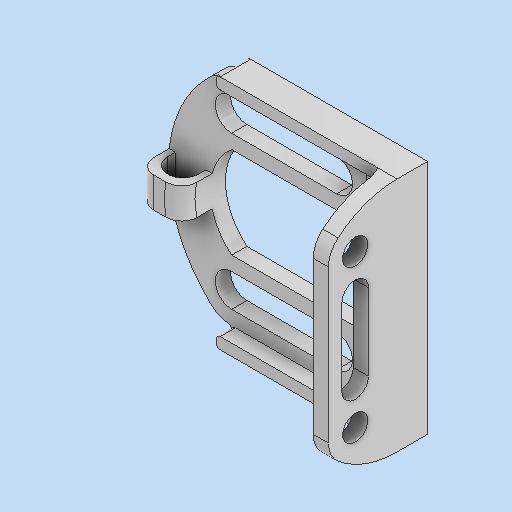
# Autodesk Inventor part: X-Gantry Enstop Mount
Saved by Autodesk Inventor 2023.2 (Build 272271000, 271)
## iProperties
Created: 2024-02-13
Part Number: X-Gantry Enstop Mount
Material: Generisch
Document SubType Name: Modeling
Designer: Nils Bade
Density: 1 g/cm^3
Appearance: Resin-3D-Druck
Description: Fertigung
Auf Bestellliste: True
Author: Nils Bade
Autodesk Inventor part; units mm, degrees
ref_plane "YZ Plane" through (0, 0, 0) normal (1, 0, 0) x (0, 1, 0)
sketch "S-Schiene" plane through (0, 0, 0) normal (0, 0, 1) x (1, 0, 0)
  line L0 (-30.84, 0) -> (5.14, 0)
  line L1 (0, -9.1) -> (0, 19.6)
  circle A0 centre (-8.51163, 10) radius 2.15 construction
  circle A1 centre (-8.51163, 10) radius 3.5 construction
  line L2 (-4, 10) -> (-21.7, 10) construction
  line L3 (-4, 12.15) -> (-21.7, 12.15)
  line L4 (-21.7, 7.85) -> (-4, 7.85)
  arc A2 (-4, 7.85) -> (-4, 12.15) centre (-4, 10) ccw
  arc A3 (-21.7, 12.15) -> (-21.7, 7.85) centre (-21.7, 10) ccw
  line L5 (-4, 10) -> (-21.7, 10) construction
  line L6 (0, 14) -> (-21.7, 14)
  line L7 (-21.7, 6) -> (0, 6)
  arc A4 (-4, 6) -> (-4, 14) centre (-4, 10) ccw construction
  arc A5 (-21.7, 14) -> (-21.7, 6) centre (-21.7, 10) ccw
  circle A6 centre (-7.766156, 0) radius 5 construction
  line L8 (-21.7, 10) -> (-8, 10) construction
  line L9 (-21.7, 7.849114) -> (-8, 7.849114)
  line L10 (-8, 12.150886) -> (-21.7, 12.150886)
  arc A7 (-21.7, 12.150886) -> (-21.7, 7.849114) centre (-21.7, 10) ccw
  arc A8 (-8, 7.849114) -> (-8, 12.150886) centre (-8, 10) ccw
  line L11 (0, 14) -> (-21.7, 14)
  line L12 (-21.7, 14) -> (-21.7, 15.5)
  line L13 (-21.7, 15.5) -> (0, 15.5)
  line L14 (0, 15.5) -> (0, 14)
  point P0 (-12.85, 10)
  point P1 (-12.85, 10)
  point P2 (0, 10)
  point P3 (-23.85, 10)
  point P4 (-1.85, 10)
  point P5 (0, 0)
  point P6 (-14.85, 10)
  point P7 (-7.938264, 12.15)
  point P8 (-7.938264, 7.85)
  point P9 (0, 15.5)
  dimension "d1" = 4.3
  dimension "d2" = 7
  dimension "d3" = 10
  dimension "d4" = 4.3
  dimension "d5" = 8
  dimension "d6" = 22
  dimension "d10" = 10
  dimension "d24" = 4
  dimension "d45" = 1.5
  constraints: 32 end point, 15 point on circle, 12 tangent, 9 centre point, 8 point on line, 6 equal length, 3 midpoint, 2 perpendicular, 1 coincident, 1 horizontal
  measures "d1" diameter of A0
  measures "d2" diameter of A1
  measures "d3" distance from line of A0.centre L0
  measures "d4" diameter of A3
  measures "d5" diameter of A5
  measures "d6" distance of point (-23.85, 10) point (-1.85, 10)
  measures "d10" diameter of A6
  measures "d24" distance of L2.start L8.end
  measures "d45" distance between parallel lines of L11 L13
sketch "S-Schiene outline for Ex-Schiene" plane through (0, 0, 0) normal (0, 0, 1) x (1, 0, 0)
  arc A0 (-21.7, 14) -> (-21.7, 6) centre (-21.7, 10) ccw
  line L0 (-21.7, 6) -> (0, 6)
  line L1 (0, 6) -> (0, 14)
  line L2 (0, 14) -> (-21.7, 14)
  line L3 (-21.7, 12.15) -> (-7.938264, 12.15)
  arc A1 (-7.938264, 12.15) -> (-7.938264, 7.85) centre (-8, 10) cw
  line L4 (-7.938264, 7.85) -> (-21.7, 7.85)
  arc A2 (-21.7, 7.85) -> (-21.7, 12.15) centre (-21.7, 10) cw
extrude "Ex-Schiene" add sketch "S-Schiene outline for Ex-Schiene" along normal blind 2
sketch "S-Schiene outline for Ex-Biegesteifigkeit" plane through (0, 0, 0) normal (0, 0, 1) x (1, 0, 0)
  line L0 (-21.7, 15.5) -> (-21.7, 14)
  line L1 (0, 15.5) -> (-21.7, 15.5)
  line L2 (0, 14) -> (0, 15.5)
  line L3 (-21.7, 14) -> (0, 14)
extrude "Ex-Biegesteifigkeit" add sketch "S-Schiene outline for Ex-Biegesteifigkeit" along normal blind 4
sketch "S-Front" plane through (0, 0, 0) normal (1, 0, 0) x (0, 1, 0)
  circle A0 centre (10, 9.5) radius 1.65
  circle A1 centre (10, 9.5) radius 3
  line L0 (6, 2) -> (14, 2) construction
  line L1 (0, 9.5) -> (5.032699, 9.5) construction
  line L2 (0, 7.75) -> (5.032699, 7.75)
  line L3 (5.032699, 11.25) -> (0, 11.25)
  arc A2 (0, 11.25) -> (0, 7.75) centre (0, 9.5) ccw construction
  arc A3 (5.032699, 7.75) -> (5.032699, 11.25) centre (5.032699, 9.5) ccw
  line L4 (0, 15.6) -> (0, -2.6)
  line L5 (0, 9.5) -> (10, 9.5) construction
  line L6 (0, 6) -> (10, 6) construction
  line L7 (10, 13) -> (0, 13)
  arc A4 (0, 13) -> (0, 6) centre (0, 9.5) ccw construction
  arc A5 (10, 6) -> (10, 13) centre (10, 9.5) ccw
  line L8 (14, 0) -> (14, 2)
  line L9 (6, 0) -> (14, 0)
  line L10 (6, 0) -> (6, 2)
  line L11 (6, 0) -> (0, 0)
  line L12 (14, 2) -> (6, 2)
  line L13 (15.5, 0) -> (15.5, 4)
  arc A6 (15.5, 4) -> (12.682482, 11.748175) centre (3.4375, 4) ccw
  line L14 (6, 0) -> (15.5, 0)
  line L15 (15.5, 0) -> (15.5, 4)
  line L16 (14, 4) -> (15.5, 4)
  line L17 (14, 2) -> (14, 4)
  line L18 (6, 2) -> (14, 2)
  line L19 (6, 0) -> (6, 2)
  point P0 (2.51635, 9.5)
  point P1 (5, 9.5)
  point P2 (0, 13)
  dimension "d11" = 3.3
  dimension "d13" = 6
  dimension "d15" = 3.5
  dimension "d16" = 7
  dimension "d23" = 9.5
  constraints: 18 end point, 11 point on circle, 10 tangent, 7 centre point, 2 coincident, 2 midpoint, 2 parallel, 1 perpendicular, 1 point on line
  measures "d11" diameter of A0
  measures "d13" diameter of A1
  measures "d15" diameter of A3
  measures "d16" diameter of A5
  measures "d23" distance from line of L9 A0.centre
sketch "S-Front outline for Ex-Front" plane through (0, 0, 0) normal (1, 0, 0) x (0, 1, 0)
  line L0 (6, 0) -> (14, 0)
  line L1 (0, 0) -> (6, 0)
  line L2 (14, 0) -> (15.5, 0)
  line L3 (0, 7.75) -> (0, 0)
  line L4 (15.5, 0) -> (15.5, 4)
  line L5 (5.032699, 7.75) -> (0, 7.75)
  arc A0 (15.5, 4) -> (12.682482, 11.748175) centre (3.4375, 4) ccw
  arc A1 (5.032699, 11.25) -> (5.032699, 7.75) centre (5.032699, 9.5) cw
  arc A2 (12.682482, 11.748175) -> (10, 13) centre (10, 9.5) ccw
  line L6 (0, 11.25) -> (5.032699, 11.25)
  line L7 (10, 13) -> (0, 13)
  line L8 (0, 13) -> (0, 11.25)
  circle A3 centre (10, 9.5) radius 1.65
extrude "Ex-Front" add sketch "S-Front outline for Ex-Front" along normal blind 2
fillet "Rundung-4mm" radius 4 2 edges at (0, 6, 1) (0, 10, 2)
extrude "Ex-SchraubenkopfEinlasss" [suppressed]
mirror "Spiegeln2" about plane through (0, 0, 0) normal (0, 1, 0)
ref_plane "E-Slide1" through (-21.7, 10, 0) normal (0, -1, 0) x (1, 0, 0)
ref_plane "E-slide2" through (-21.7, -10, 0) normal (0, -1, 0) x (1, 0, 0)
sketch "S-Extension" plane through (0, 0, 0) normal (0, 0, 1) x (1, 0, 0)
  arc A0 (-21.7, 14) -> (-21.7, 6) centre (-21.7, 10) ccw
  arc A1 (-21.7, -6) -> (-21.7, -14) centre (-21.7, -10) ccw
  arc A2 (-21.7, -6) -> (-21.7, -14) centre (-21.7, -10) ccw
  arc A3 (-21.7, 6) -> (-21.7, -6) centre (-16.705119, 0) ccw
  arc A4 (-21.7, 14) -> (-21.7, 6) centre (-21.7, 10) ccw
  arc A5 (-24.406352, 12.945447) -> (-24.445645, -12.908854) centre (-12.261257, -0.000191) ccw
  line L0 (-24.251564, 2) -> (-29.899061, 2)
  line L1 (-36.038087, 0) -> (6.006348, 0) construction
  line L2 (-29.899104, -2) -> (-24.251564, -2)
  point P0 (0, 0)
  point P1 (-24.484334, 12.871843)
  point P2 (-24.445645, -12.908854)
  dimension "d34" = 2
  dimension "d36" = 2
  constraints: 10 point on circle, 4 end point, 2 centre point, 2 horizontal, 1 tangent
  measures "d34" distance between parallel lines of L1 L0
  measures "d36" distance between parallel lines of L2 L1
sketch "S-Extension outline for Ex-Extension1" plane through (0, 0, 0) normal (0, 0, 1) x (1, 0, 0)
  arc A0 (-21.7, -6) -> (-21.7, 6) centre (-16.705119, 0) cw
  arc A1 (-24.445645, -12.908854) -> (-21.7, -6) centre (-21.7, -10) cw
  arc A2 (-24.484334, 12.871843) -> (-24.445645, -12.908854) centre (-12.261257, -0.000191) ccw
  arc A3 (-21.7, 6) -> (-24.484334, 12.871843) centre (-21.7, 10) cw
extrude "Ex-Extension1" add sketch "S-Extension outline for Ex-Extension1" along normal blind 2
sketch "S-Extension outline for Ex-Extension2" plane through (0, 0, 0) normal (0, 0, 1) x (1, 0, 0)
  line L0 (-29.899104, -2) -> (-24.251564, -2)
  arc A0 (-29.899061, 2) -> (-29.899104, -2) centre (-12.261257, -0.000191) ccw
  line L1 (-24.251564, 2) -> (-29.899061, 2)
  arc A1 (-24.251564, -2) -> (-24.251564, 2) centre (-16.705119, 0) cw
extrude "Ex-Extension2" add sketch "S-Extension outline for Ex-Extension2" along normal blind 6
sketch "Skizze5" plane through (-29.899104, -2, 2) normal (0, -1, 0) x (1, 0, 0)
  line L0 (5.64754, 0) -> (0, 0)
  line L1 (5.64754, 0) -> (5.64754, 4)
  line L2 (0, 4) -> (5.64754, 4)
  line L3 (0, 0) -> (0, 4)
  line L4 (5.41477, 0) -> (0.000043, 0)
  line L5 (0.82377, 0) -> (4.82377, 0)
  line L6 (4.82377, 0) -> (4.82377, 3)
  line L7 (4.82377, 3) -> (0.82377, 3)
  line L8 (0.82377, 3) -> (0.82377, 0)
  line L9 (0, 4) -> (5.64754, 4) construction
  line L10 (2.82377, 4) -> (2.82377, 0) construction
  point P0 (29.899104, -2)
  point P1 (2.82377, 3)
  point P2 (0.82377, 0)
  point P3 (4.82377, 0)
  dimension "d40" = 4
  dimension "d41" = 3
  constraints: 10 end point, 3 midpoint, 2 parallel, 2 point on line, 1 horizontal, 1 perpendicular
  measures "d40" distance between parallel lines of L6 L8
  measures "d41" distance between parallel lines of L0 L7
sketch "Skizze5 outline for Ex-Extension3" plane through (-29.899104, -2, 2) normal (0, -1, 0) x (1, 0, 0)
  line L0 (4.82377, 3) -> (0.82377, 3)
  line L1 (4.82377, 0) -> (4.82377, 3)
  line L2 (0.82377, 0) -> (4.82377, 0)
  line L3 (0.82377, 3) -> (0.82377, 0)
extrude "Ex-Extension3" cut sketch "Skizze5 outline for Ex-Extension3" against normal up to surface (4 mm away)
fillet "Rundung-2mm" radius 2 4 edges at (-25.0753, 0, 5) (-29.0753, 0, 5) (-24.5121, 0, 6) (-30.0121, 0, 6)
fillet "Rundung-0.5mm" radius 0.5 6 edges at (-21.7, 14, 1) (-21.7, 15.5, 2) (-21.7, 14, 3) (-21.7, -14, 3) (-21.7, -14, 1) (-21.7, -15.5, 2)
equation "\"d36\" = d34"
